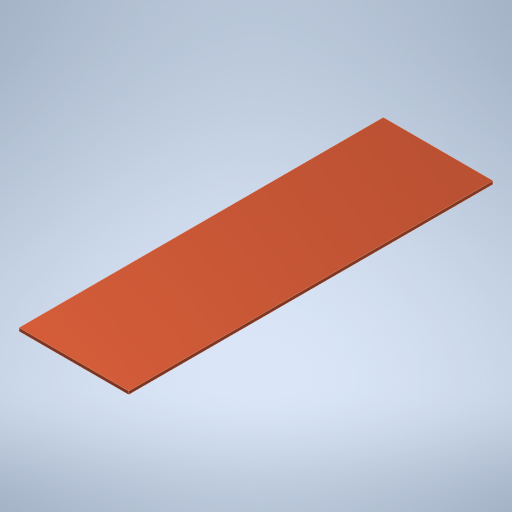
# Autodesk Inventor part: top_v2
Saved by Autodesk Inventor 2023 (Build 270158000, 158)
## iProperties
Created: 2022-09-23
Part Number: top_v2
Material: Generic
Document SubType Name: Modeling
Designer: Desmond
Density: 1 g/cm^3
Appearance: Copper - Satin
Author: Desmond
Autodesk Inventor part; units mm, degrees
ref_plane "YZ Plane" through (0, 0, 0) normal (1, 0, 0) x (0, 1, 0)
ref_plane "XZ Plane" through (0, 0, 0) normal (0, 1, 0) x (-1, 0, 0)
ref_plane "XY Plane" through (0, 0, 0) normal (0, 0, 1) x (1, 0, 0)
sketch "Sketch1" plane through (0, 0, 0) normal (0, 1, 0) x (-1, 0, 0)
  line L0 (0, 0) -> (56, 0)
  line L1 (56, 0) -> (56, -186)
  line L2 (56, -186) -> (0, -186)
  line L3 (0, -186) -> (0, 0)
  dimension "d0" = 56
  dimension "d1" = 186
  constraints: 8 end point, 2 parallel, 1 horizontal, 1 perpendicular
  measures "d0" distance of L1.end L2.end
  measures "d1" distance of L0.end L1.end
extrude "Extrusion1" add sketch "Sketch1" along normal blind 1.6
body "Solid1"
